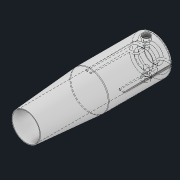
# Autodesk Inventor part: grip
Saved by Autodesk Inventor 2022 (Build 260153000, 153)
## iProperties
Created: 2024-04-29
Part Number: grip
Material: 一般
Document SubType Name: Modeling
Designer: gisen
Density: 1 g/cm^3
Appearance: 既定
Author: gisen
Autodesk Inventor part; units mm, degrees
ref_plane "YZ Plane" through (0, 0, 0) normal (1, 0, 0) x (0, 1, 0)
ref_plane "XY Plane" through (0, 0, 0) normal (0, 0, 1) x (1, 0, 0)
sketch "スケッチ1" plane through (0, 0, 0) normal (0, 1, 0) x (-1, 0, 0)
  line L0 (-10.7, 92) -> (-11, 0)
  line L1 (-11, 0) -> (0, 0)
  line L2 (0, 0) -> (0, -8)
  line L3 (0, -8) -> (-15, -8) construction
  line L4 (-15, -8) -> (-15, 42) construction
  line L5 (-14.9723, 42.7435) -> (-11.3, 92)
  arc A0 (-14.9723, 42.7435) -> (-15, 42) centre (-5, 42) ccw
  circle A1 centre (0, -2) radius 1.65 construction
  circle A2 centre (0, -2) radius 6 construction
  circle A3 centre (-11, 0) radius 4 construction
  line L6 (-15, 42) -> (-15, 0)
  line L7 (-2.112, -7.616) -> (-12.408, -3.744) construction
  arc A4 (-15, 0) -> (-12.408, -3.744) centre (-11, 0) ccw construction
  arc A5 (-2.112, -7.616) -> (0, -8) centre (0, -2) ccw construction
  line L8 (0, -28.1143) -> (0, 112.019) projected
  line L9 (-15, 0) -> (-15, -8)
  line L10 (-15, -8) -> (0, -8)
  line L11 (-11.3, 92) -> (-10.7, 92)
  dimension "d1" = 10
  dimension "d3" = 15
  dimension "d5" = 8
  dimension "d6" = 50
  dimension "d7" = 3.3
  dimension "d8" = 2
  dimension "d29" = 0.6
  dimension "d30" = 11
  dimension "d31" = 10.7
  dimension "d32" = 92
  constraints: 22 end point, 10 point on circle, 8 tangent, 6 centre point, 4 coincident, 3 perpendicular, 2 horizontal, 2 point on line, 1 collinear
  measures "d1" radius of A0
  measures "d3" distance between parallel lines of L4 L2
  measures "d5" distance between parallel lines of L3 L1
  measures "d6" distance of L3.end L4.end
  measures "d7" diameter of A1
  measures "d8" distance from line of L1 A1.centre
  measures "d29" distance of L5.end L0.start
  measures "d30" distance from line of L0.end L8
  measures "d31" distance from line of L8 L0.start
  measures "d32" distance from line of L1 L0.start
revolve "回転1" add sketch "スケッチ1" angle 360 about axis through (0, 0, -10) along (0, 0, 1)
sketch "スケッチ2" plane through (0, 0, 0) normal (0, 1, 0) x (-1, 0, 0)
  circle A0 centre (0, -2) radius 1.65
  line L0 (11, 0) -> (-11, 0) projected
  point P0 (0, 0)
  dimension "d10" = 3.3
  dimension "d23" = 2
  constraints: 1 centre point, 1 coincident
  measures "d10" diameter of A0
  measures "d23" distance from line of point (0, -2) L0
extrude "押し出し1" cut sketch "スケッチ2" along normal through all both and the other way through all
sketch "スケッチ3" plane through (0, 0, 0) normal (1, 0, 0) x (0, 1, 0)
  line L0 (0, -10) -> (0, 0) construction
  line L1 (1, -10) -> (-1, -10)
  line L2 (-1, -10) -> (-0.4, 30.006)
  line L3 (0.4, 30.006) -> (1, -10)
  arc A0 (0.4, 30.006) -> (-0.4, 30.006) centre (0, 30) ccw
  dimension "d13" = 0.4
  dimension "d14" = 2
  dimension "d15" = 40
  constraints: 8 end point, 2 point on circle, 2 tangent, 1 centre point, 1 equal length, 1 horizontal, 1 midpoint, 1 vertical
  measures "d13" radius of A0
  measures "d14" distance of L1.start L1.end
  measures "d15" distance from line of L1 A0.centre
extrude "押し出し2" cut sketch "スケッチ3" along normal through all both and the other way through all
ref_plane "作業平面1" through (0, 12, 0) normal (0, 1, 0) x (-1, 0, 0)
ref_plane "作業平面2" through (0, -12, 0) normal (0, 1, 0) x (-1, 0, 0)
sketch "スケッチ4" plane through (0, 12, 0) normal (0, 1, 0) x (-1, 0, 0)
  circle A0 centre (0, -2) radius 2.9
  circle A1 centre (0, -2) radius 1.65 construction
  dimension "d20" = 5.8
  constraints: 1 centre point, 1 concentric
  measures "d20" diameter of A0
extrude "押し出し3" cut sketch "スケッチ4" along normal through all
sketch "スケッチ5" plane through (0, -12, 0) normal (0, 1, 0) x (-1, 0, 0)
  line L0 (-1.5877, -4.75) -> (-3.1754, -2)
  line L1 (-3.1754, -2) -> (-1.5877, 0.75)
  line L2 (-1.5877, 0.75) -> (1.5877, 0.75)
  line L3 (1.5877, 0.75) -> (3.1754, -2)
  line L4 (3.1754, -2) -> (1.5877, -4.75)
  line L5 (1.5877, -4.75) -> (-1.5877, -4.75)
  point P0 (0, 0)
  point P1 (0, -2)
  point P2 (0, -2)
  dimension "d24" = 5.5
  constraints: 12 end point, 1 coincident, 1 horizontal, 13 other
  measures "d24" distance between parallel lines of L5 L2
extrude "押し出し4" cut sketch "スケッチ5" against normal through all
fillet "フィレット1" radius 2 2 edges at (0, 15, -8) (0, -15, -8)
chamfer "面取り1" [suppressed]
sketch "スケッチ6" plane through (0, 0, -8) normal (0, 0, -1) x (-1, 0, 0)
  circle A0 centre (0, 0) radius 6
  dimension "d37" = 12
  constraints: 1 centre point, 1 coincident
  measures "d37" diameter of A0
extrude "押し出し5" cut sketch "スケッチ6" against normal through all
chamfer "面取り2" distance 1.5 angle 45 4 edges at (0, -6, -8) (0, -6, 0) (0, 6, 0) (0, 6, -8)
equation "\"d19\" = -d18"
equation "\"d18\" = 12"
